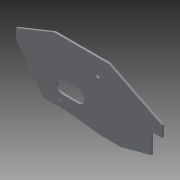
# Autodesk Inventor part: ShooterMountRight_NERDS
Saved by Autodesk Inventor 2014 (Build 180170000, 170)
## iProperties
Created: 2016-01-30
Part Number: ShooterMountRight_NERDS
Material: Generic
Document SubType Name: Modeling
Designer: bermudezr
Density: 1 g/cm^3
Appearance: Default
Author: bermudezr
Autodesk Inventor part; units mm, degrees
ref_plane "YZ Plane" through (0, 0, 0) normal (1, 0, 0) x (0, 1, 0)
ref_plane "XZ Plane" through (0, 0, 0) normal (0, 1, 0) x (-1, 0, 0)
ref_plane "XY Plane" through (0, 0, 0) normal (0, 0, 1) x (1, 0, 0)
sketch "Sketch1" plane through (0, 0, 0) normal (0, 0, 1) x (1, 0, 0)
  line L0 (-84.0821, 192.7052) -> (642.9929, 192.7052)
  line L1 (642.9929, 192.7052) -> (642.9929, -137.4948)
  line L2 (642.9929, -137.4948) -> (-84.0821, -137.4948)
  line L3 (-84.0821, -137.4948) -> (-84.0821, 192.7052)
  circle A0 centre (131.8179, -86.6948) radius 4.7625
  circle A1 centre (323.5837, 116.5052) radius 12.7
  line L4 (642.9929, -137.4948) -> (592.1929, -137.4948)
  line L5 (592.1929, -137.4948) -> (592.1929, -73.9948)
  line L6 (592.1929, -73.9948) -> (642.9929, -73.9948)
  line L7 (642.9929, -73.9948) -> (642.9929, -137.4948)
  line L8 (642.9929, 192.7052) -> (592.6352, 192.7052)
  line L9 (642.9929, 2.2052) -> (642.9929, 192.7052)
  line L10 (-84.0821, 53.0052) -> (5.7204, 53.0052) construction
  line L11 (-84.0821, 65.7052) -> (68.3179, -137.4948)
  line L12 (595.3679, 192.7052) -> (595.3679, 2.2052)
  line L13 (595.3679, 2.2052) -> (642.9929, 2.2052)
  point P0 (0, 0)
  dimension "d0" = 727.075
  dimension "d2" = 9.525
  dimension "d3" = 25.4
  dimension "d4" = 215.9
  dimension "d5" = 279.4
  dimension "d14" = 152.4
  dimension "d15" = 203.2
  dimension "d16" = 330.2
  dimension "d17" = 63.5
  dimension "d19" = 50.8
  dimension "d20" = 139.7
  dimension "d21" = 50.8
  dimension "d22" = 254
  constraints: 28 end point, 5 parallel, 5 point on line, 4 horizontal, 3 perpendicular, 2 centre point
  measures "d0" distance of L1.end L2.end
  measures "d2" diameter of A0
  measures "d3" diameter of A1
  measures "d4" distance from line of L3 A0.centre
  measures "d5" distance of A1.centre A0.centre
  measures "d14" distance from line of L3 L11.end
  measures "d15" distance from line of L2 L11.start
  measures "d16" distance between parallel lines of L2 L0
  measures "d17" distance between parallel lines of L6 L2
  measures "d19" distance of L5.end L6.end
  measures "d20" distance between parallel lines of L13 L4
  measures "d21" distance from line of L2 A0.centre
  measures "d22" distance from line of L2 A1.centre
extrude "Extrusion1" add sketch "Sketch1" along normal blind 9.525 contours L0 L12 L13 L1 L6 L5 L2 L11 L3
sketch "Sketch2" plane through (0, 0, 9.525) normal (0, 0, 1) x (1, 0, 0)
  line L0 (595.3679, 2.2052) -> (595.3679, 192.7052) projected
  line L1 (595.3679, 192.7052) -> (-84.0821, 192.7052) projected
  line L2 (-84.0821, 192.7052) -> (-84.0821, 65.7052) projected
  line L3 (68.3179, -137.4948) -> (592.1929, -137.4948) projected
  line L4 (592.1929, -137.4948) -> (592.1929, -73.9948) projected
  line L5 (-84.0821, 116.5052) -> (106.4179, 192.7052)
  line L6 (379.4679, 192.7052) -> (646.1679, 59.3552)
  line L7 (595.3679, 84.7552) -> (595.3679, 192.7052)
  point P0 (0, 0)
  dimension "d25" = 190.5
  dimension "d26" = 50.8
  dimension "d28" = 196.85
  dimension "d30" = 53.975
  dimension "d31" = 212.725
  constraints: 6 end point, 5 point on line, 1 collinear
  measures "d25" distance from line of L2 L5.end
  measures "d26" distance of L2.end L5.start
  measures "d28" distance from line of L3 L6.end
  measures "d30" distance from line of L6.end L4
  measures "d31" distance from line of L6.start L4
extrude "Extrusion2" cut sketch "Sketch2" against normal blind 25.4
sketch "Sketch3" plane through (0, 0, 9.525) normal (0, 0, 1) x (1, 0, 0)
  line L0 (592.1929, -137.4948) -> (740.2432, -137.4948)
  line L1 (740.2432, -137.4948) -> (740.2432, 103.8052)
  line L2 (740.2432, 103.8052) -> (592.1929, 103.8052)
  line L3 (592.1929, 103.8052) -> (592.1929, -137.4948)
  point P0 (0, 0)
  constraints: 8 end point, 2 parallel, 1 horizontal, 1 perpendicular
extrude "Extrusion3" cut sketch "Sketch3" against normal blind 25.4
sketch "Sketch4" plane through (0, 0, 9.525) normal (0, 0, 1) x (1, 0, 0)
  line L0 (592.1929, -137.4948) -> (592.1929, 86.3427) projected
  line L1 (592.1929, 86.3427) -> (379.4679, 192.7052) projected
  line L2 (68.3179, -137.4948) -> (592.1929, -137.4948) projected
  line L3 (592.1929, 86.3427) -> (646.1679, 59.3552)
  line L4 (646.1679, 59.3552) -> (646.1679, 40.3052)
  line L5 (646.1679, 40.3052) -> (592.1929, 40.3052)
  point P0 (0, 0)
  dimension "d37" = 53.975
  dimension "d38" = 19.05
  constraints: 6 end point, 2 perpendicular, 1 collinear, 1 point on line
  measures "d37" distance from line of L3.end L0
  measures "d38" distance of L3.end L4.end
extrude "Extrusion4" add sketch "Sketch4" against normal blind 9.525
sketch "Sketch5" plane through (0, 0, 9.525) normal (0, 0, 1) x (1, 0, 0)
  line L0 (592.1929, 40.3052) -> (646.1679, 40.3052)
  line L1 (646.1679, 40.3052) -> (646.1679, 5.3802)
  line L2 (646.1679, 5.3802) -> (592.1929, 5.3802)
  line L3 (592.1929, 5.3802) -> (592.1929, 40.3052)
  point P0 (0, 0)
  dimension "d41" = 34.925
  constraints: 8 end point, 2 parallel, 1 horizontal, 1 perpendicular
  measures "d41" distance of L0.end L1.end
extrude "Extrusion5" add sketch "Sketch5" against normal blind 9.525
sketch "Sketch6" plane through (0, 0, 9.525) normal (0, 0, 1) x (1, 0, 0)
  line L0 (-84.0821, 65.7052) -> (68.3179, -137.4948)
  line L1 (68.3179, -137.4948) -> (592.1929, -137.4948)
  line L2 (592.1929, -137.4948) -> (592.1929, 40.3052)
  line L3 (147.7945, 9.1902) -> (225.2645, 9.1902)
  line L4 (341.7489, -137.4948) -> (170.3104, -117.1748)
  line L5 (170.3104, -117.1748) -> (53.0779, -117.1748)
  line L6 (68.3179, -137.4948) -> (592.1929, -137.4948) projected
  line L7 (592.1929, -96.6594) -> (439.7929, -137.4948)
  line L8 (439.7929, -137.4948) -> (592.1929, -137.4948)
  line L9 (592.1929, -137.4948) -> (592.1929, -96.6594)
  point P0 (0, 0)
  point P1 (0, 0)
  dimension "d47" = 20.32
  dimension "d50" = 152.4
  dimension "d53" = 173.24
  dimension "d54" = 165
  dimension "d55" = 98.044
  constraints: 18 end point, 4 point on line, 2 collinear, 1 parallel
  measures "d47" distance between parallel lines of L1 L5
  measures "d50" distance from line of L2 L7.end
  measures "d53" angle of L4 L1
  measures "d54" angle of L1 L7
  measures "d55" distance of L7.end L4.start
extrude "Extrusion7" cut sketch "Sketch6" against normal blind 25.4
sketch "Sketch7" plane through (0, 0, 0) normal (0, 0, -1) x (-1, 0, 0)
  line L0 (-68.3179, -137.4948) -> (-592.1929, -137.4948)
  line L1 (84.0821, 192.7052) -> (84.0821, 65.7052)
  circle A0 centre (-147.7945, -23.1948) radius 32.385
  circle A1 centre (-225.2645, -23.1948) radius 32.385
  line L2 (-225.2645, 9.1902) -> (-147.7945, 9.1902)
  line L3 (-225.2645, -55.5798) -> (-147.7945, -55.5798)
  circle A2 centre (-323.5837, 116.5052) radius 12.7
  line L4 (-595.3679, 192.7052) -> (-595.3679, 2.2052)
  line L5 (-595.3679, 2.2052) -> (-642.9929, 2.2052)
  line L6 (-642.9929, -73.9948) -> (-642.9929, 2.2052)
  line L7 (-642.9929, -73.9948) -> (-592.1929, -73.9948)
  line L8 (-592.1929, -73.9948) -> (-592.1929, -137.4948)
  line L9 (84.0821, 65.7052) -> (-68.3179, -137.4948)
  line L10 (-595.3679, 192.7052) -> (84.0821, 192.7052)
  circle A3 centre (-131.8179, -86.6948) radius 4.7625
  point P0 (0, 0)
  point P1 (0, 0)
  dimension "d56" = 64.77
  dimension "d57" = 231.8766
  dimension "d58" = 114.3
  dimension "d59" = 64.77
  dimension "d60" = 77.47
  constraints: 22 end point, 4 centre point, 4 point on circle, 4 tangent
  measures "d56" diameter of A0
  measures "d57" distance from line of L1 A0.centre
  measures "d58" distance from line of A0.centre L0
  measures "d59" diameter of A1
  measures "d60" distance of A0.centre A1.centre
extrude "Extrusion8" cut sketch "Sketch7" against normal blind 25.4 contours A0 | A0 L3 A1 L2 | A1
body "Solid1"
